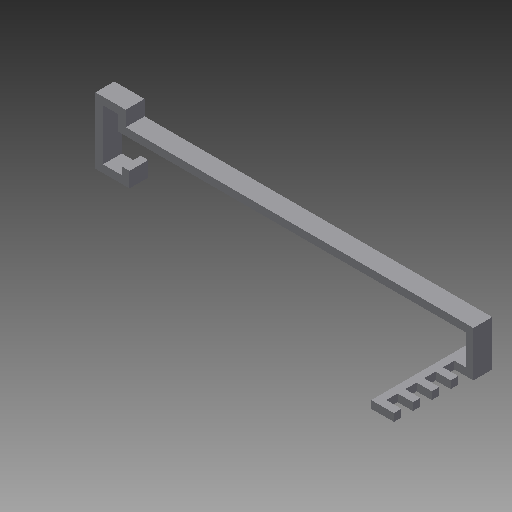
# Autodesk Inventor part: Steunbalk boven
Saved by Autodesk Inventor 2018.3 (Build 223284000, 284)
## iProperties
Created: 2020-11-17
Part Number: Steunbalk boven
Material: Generic
Document SubType Name: Modeling
Designer: daanv
Density: 1 g/cm^3
Appearance: Default
Author: daanv
Autodesk Inventor part; units mm, degrees
ref_plane "YZ Plane" through (0, 0, 0) normal (1, 0, 0) x (0, 1, 0)
ref_plane "XZ Plane" through (0, 0, 0) normal (0, 1, 0) x (-1, 0, 0)
ref_plane "XY Plane" through (0, 0, 0) normal (0, 0, 1) x (1, 0, 0)
sketch "Sketch1" plane through (0, 0, 0) normal (0, 0, 1) x (1, 0, 0)
  line L0 (0, 0) -> (6, 0)
  line L1 (6, 0) -> (6, 2)
  line L2 (6, 2) -> (0, 2)
  line L3 (0, 2) -> (0, 0)
  dimension "d0" = 6
  dimension "d1" = 2
  constraints: 8 end point, 2 parallel, 1 horizontal, 1 perpendicular
  measures "d0" distance of L2.end L1.end
  measures "d1" distance of L1.end L0.end
extrude "Extrusion1" add sketch "Sketch1" along normal blind 5
sketch "Sketch2" plane through (0, 0, 0) normal (-1, 0, 0) x (0, 0, 1)
  line L0 (0, 2) -> (0, 0) projected
  line L1 (0, 0) -> (5, 0) projected
  line L2 (5, 2) -> (5, 0) projected
  line L3 (0, 2) -> (5, 2) projected
extrude "Extrusion2" add sketch "Sketch2" along normal blind 2
sketch "Sketch3" plane through (6, 0, 0) normal (0, -1, 0) x (1, 0, 0)
  line L0 (-8, 5) -> (-6, 5)
  line L1 (-6, 5) -> (-6, 0)
  line L2 (-6, 0) -> (-8, 0)
  line L3 (-8, 0) -> (-8, 5)
  constraints: 8 end point, 2 parallel, 1 horizontal, 1 perpendicular
extrude "Extrusion3" add sketch "Sketch3" along normal blind 10.5
sketch "Sketch5" plane through (6, 0, 0) normal (0, -1, 0) x (1, 0, 0)
  line L0 (0, 5) -> (-8, 5) projected
  line L1 (0, 0) -> (-8, 0) projected
  line L2 (0, 5) -> (-2, 5)
  line L3 (-2, 5) -> (-2, 0)
  line L4 (-2, 0) -> (0, 0)
  line L5 (0, 0) -> (0, 5)
  constraints: 8 end point, 2 parallel, 1 horizontal, 1 perpendicular, 1 point on line
extrude "Extrusion5" add sketch "Sketch5" along normal blind 4
sketch "Sketch6" plane through (6, 2, 5) normal (1, 0, 0) x (0, 0, -1)
  line L0 (0, -6) -> (5, -6) projected
  line L1 (5, -2) -> (5, -12.5) projected
  line L2 (0, -6) -> (5, -6)
  line L3 (5, -6) -> (5, -4)
  line L4 (5, -4) -> (0, -4)
  line L5 (0, -4) -> (0, -6)
  dimension "d13" = 2
  constraints: 8 end point, 2 parallel, 1 horizontal, 1 perpendicular, 1 point on line
  measures "d13" distance of L3.end L2.end
extrude "Extrusion6" add sketch "Sketch6" along normal blind 89.93
sketch "Sketch7" plane through (95.93, 2, 5) normal (1, 0, 0) x (0, 0, -1)
  line L0 (0, -6) -> (5, -6) projected
  line L1 (5, -6) -> (5, -4) projected
  line L2 (5, -4) -> (0, -4) projected
  line L3 (0, -4) -> (0, -6) projected
  point P0 (5, -2)
extrude "Extrusion7" add sketch "Sketch7" along normal blind 2
sketch "Sketch8" plane through (6, -4, 0) normal (0, -1, 0) x (1, 0, 0)
  line L0 (-2, 0) -> (91.93, 0) projected
  line L1 (91.93, 5) -> (89.93, 5)
  line L2 (89.93, 5) -> (89.93, 0)
  line L3 (89.93, 0) -> (91.93, 0)
  line L4 (91.93, 0) -> (91.93, 5)
  point P0 (-6, 0)
  dimension "d18" = 2
  constraints: 8 end point, 2 parallel, 1 horizontal, 1 perpendicular, 1 point on line
  measures "d18" distance of L3.end L2.end
extrude "Extrusion8" add sketch "Sketch8" along normal blind 10
sketch "Sketch9" plane through (6, -10.5, 0) normal (0, -1, 0) x (1, 0, 0)
  line L0 (-6, 0) -> (-6, 5) projected
  line L1 (-6, 5) -> (-8, 5) projected
  line L2 (-8, 5) -> (-8, 0) projected
  line L3 (-8, 0) -> (-6, 0) projected
extrude "Extrusion9" add sketch "Sketch9" along normal blind 5
sketch "Sketch10" plane through (0, 0, 5) normal (1, 0, 0) x (0, 0, -1)
  line L0 (0, 2) -> (0, -15.5) projected
  line L1 (5, 2) -> (5, -15.5) projected
  line L2 (0, -15.5) -> (5, -15.5)
  line L3 (5, -15.5) -> (5, -13.5)
  line L4 (5, -13.5) -> (0, -13.5)
  line L5 (0, -13.5) -> (0, -15.5)
  dimension "d23" = 2
  constraints: 8 end point, 2 parallel, 1 horizontal, 1 perpendicular, 1 point on line
  measures "d23" distance of L3.end L2.end
extrude "Extrusion10" add sketch "Sketch10" along normal blind 5
sketch "Sketch11" plane through (5, 0, 5) normal (1, 0, 0) x (0, 0, -1)
  line L0 (0, -15.5) -> (5, -15.5) projected
  line L1 (5, -15.5) -> (5, -13.5) projected
  line L2 (5, -13.5) -> (0, -13.5) projected
  line L3 (0, -13.5) -> (0, -15.5) projected
  point P0 (5, 0)
extrude "Extrusion11" add sketch "Sketch11" along normal blind 2
sketch "Sketch12" plane through (0, -13.5, 5) normal (0, 1, 0) x (1, 0, 0)
  line L0 (0, 0) -> (7, 0) projected
  line L1 (7, 5) -> (5, 5)
  line L2 (5, 5) -> (5, 0)
  line L3 (5, 0) -> (7, 0)
  line L4 (7, 0) -> (7, 5)
  dimension "d28" = 2
  constraints: 8 end point, 2 parallel, 1 horizontal, 1 perpendicular, 1 point on line
  measures "d28" distance of L3.end L2.end
extrude "Extrusion12" add sketch "Sketch12" along normal blind 2
sketch "Sketch13" plane through (95.93, -4, 0) normal (-1, 0, 0) x (0, 0, 1)
  line L0 (5, 0) -> (5, -10) projected
  line L1 (0, -10) -> (5, -10)
  line L2 (5, -10) -> (5, -8)
  line L3 (5, -8) -> (0, -8)
  line L4 (0, -8) -> (0, -10)
  point P0 (0, 4)
  dimension "d31" = 2
  constraints: 8 end point, 2 parallel, 1 horizontal, 1 perpendicular, 1 point on line
  measures "d31" distance of L2.end L1.end
extrude "Extrusion13" add sketch "Sketch13" along normal blind 5
sketch "Sketch14" plane through (0, 0, 5) normal (0, 0, 1) x (1, 0, 0)
  line L0 (97.93, -14) -> (90.93, -14) projected
  line L1 (90.93, -12) -> (92.93, -12)
  line L2 (92.93, -12) -> (92.93, -14)
  line L3 (92.93, -14) -> (90.93, -14)
  line L4 (90.93, -14) -> (90.93, -12)
  dimension "d34" = 2
  constraints: 8 end point, 2 parallel, 1 horizontal, 1 perpendicular, 1 point on line
  measures "d34" distance of L2.end L3.end
extrude "Extrusion14" add sketch "Sketch14" along normal blind 5
sketch "Sketch15" plane through (92.93, -14, 5) normal (1, 0, 0) x (0, 0, -1)
  line L0 (0, 0) -> (-5, 0) projected
  line L1 (-5, 2) -> (-3, 2)
  line L2 (-3, 2) -> (-3, 0)
  line L3 (-3, 0) -> (-5, 0)
  line L4 (-5, 0) -> (-5, 2)
  point P0 (5, 14)
  dimension "d37" = 2
  constraints: 8 end point, 2 parallel, 1 horizontal, 1 perpendicular, 1 point on line
  measures "d37" distance of L2.end L3.end
extrude "Extrusion15" add sketch "Sketch15" along normal blind 4
sketch "Sketch16" plane through (0, 0, 10) normal (0, 0, 1) x (1, 0, 0)
  line L0 (90.93, -12) -> (90.93, -14) projected
  line L1 (90.93, -14) -> (96.93, -14) projected
  line L2 (95.93, -12) -> (90.93, -12) projected
  line L3 (97.93, -14) -> (92.93, -14) projected
  line L4 (90.93, -12) -> (92.93, -12)
  line L5 (92.93, -12) -> (92.93, -14)
  line L6 (92.93, -14) -> (90.93, -14)
  line L7 (90.93, -14) -> (90.93, -12)
  point P0 (0, 0)
  constraints: 8 end point, 2 parallel, 1 horizontal, 1 perpendicular
extrude "Extrusion16" add sketch "Sketch16" along normal blind 5
sketch "Sketch17" plane through (92.93, -14, 10) normal (1, 0, 0) x (0, 0, -1)
  line L0 (-5, 2) -> (-5, 0) projected
  line L1 (10, 0) -> (-5, 0) projected
  line L2 (-5, 2) -> (-3, 2)
  line L3 (-3, 2) -> (-3, 0)
  line L4 (-3, 0) -> (-5, 0)
  line L5 (-5, 0) -> (-5, 2)
  point P0 (10, 14)
  dimension "d42" = 2
  constraints: 8 end point, 2 parallel, 1 horizontal, 1 perpendicular, 1 point on line
  measures "d42" distance of L3.end L4.end
extrude "Extrusion17" add sketch "Sketch17" along normal blind 4
sketch "Sketch18" plane through (0, 0, 15) normal (0, 0, 1) x (1, 0, 0)
  line L0 (90.93, -12) -> (90.93, -14) projected
  line L1 (90.93, -12) -> (90.93, -14) projected
  line L2 (97.93, -14) -> (90.93, -14) projected
  line L3 (90.93, -12) -> (92.93, -12)
  line L4 (92.93, -12) -> (92.93, -14)
  line L5 (92.93, -14) -> (90.93, -14)
  line L6 (90.93, -14) -> (90.93, -12)
  point P0 (0, 0)
  dimension "d45" = 2
  constraints: 8 end point, 2 parallel, 1 horizontal, 1 perpendicular, 1 point on line
  measures "d45" distance of L4.end L5.end
extrude "Extrusion18" add sketch "Sketch18" along normal blind 10
sketch "Sketch19" plane through (92.93, -14, 15) normal (1, 0, 0) x (0, 0, -1)
  line L0 (15, 2) -> (-10, 2) projected
  line L1 (15, 0) -> (-10, 0) projected
  line L2 (-3, 2) -> (-5, 2)
  line L3 (-5, 2) -> (-5, 0)
  line L4 (-5, 0) -> (-3, 0)
  line L5 (-3, 0) -> (-3, 2)
  line L6 (0, 2) -> (0, 0) projected
  point P0 (15, 14)
  dimension "d48" = 2
  dimension "d51" = 3
  constraints: 8 end point, 2 parallel, 2 point on line, 1 horizontal, 1 perpendicular
  measures "d48" distance of L4.end L3.end
  measures "d51" distance between parallel lines of L6 L5
extrude "Extrusion19" add sketch "Sketch19" along normal blind 4 contours L5 L1 L3 L0
sketch "Sketch20" plane through (92.93, -14, 25) normal (1, 0, 0) x (0, 0, -1)
  line L0 (25, 2) -> (0, 2) projected
  line L1 (25, 0) -> (0, 0) projected
  line L2 (0, 2) -> (2, 2)
  line L3 (2, 2) -> (2, 0)
  line L4 (2, 0) -> (0, 0)
  line L5 (0, 0) -> (0, 2)
  point P0 (25, 14)
  dimension "d52" = 2
  constraints: 8 end point, 2 parallel, 1 horizontal, 1 perpendicular, 1 point on line
  measures "d52" distance of L3.end L4.end
extrude "Extrusion20" add sketch "Sketch20" along normal blind 4
body "Solid1"
